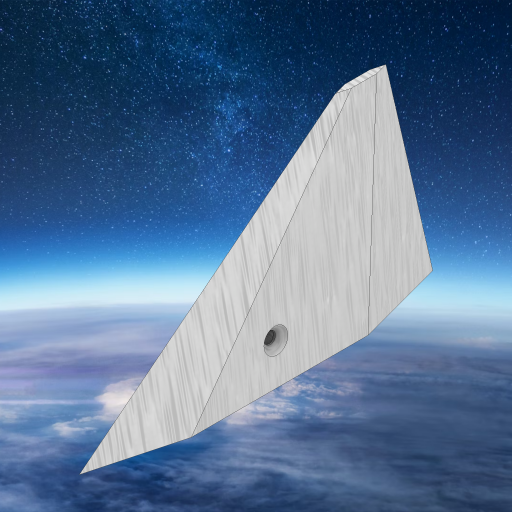
# Autodesk Inventor part: canard
Saved by Autodesk Inventor 2023 (Build 270158000, 158)
## iProperties
Created: 2022-11-29
Part Number: canard
Material: Aluminum 7075
Document SubType Name: Modeling
Designer: 310611102
Density: 2.81 g/cm^3
Appearance: Satin - Brushed Heavy
Mass: 264.064 g
Surface Area: 174.305 cm^2
Volume: 93.9731 cm^3
Author: 310611102
Autodesk Inventor part; units mm, degrees
ref_plane "XY Plane" through (0, 0, 0) normal (0, 0, 1) x (1, 0, 0)
sketch "草圖1" plane through (0, 0, 0) normal (1, 0, 0) x (0, 1, 0)
  line L0 (0, 0) -> (0, -140)
  line L1 (0, -140) -> (80, -121.4423)
  line L2 (80, -121.4423) -> (80, -101.4423)
  line L3 (80, -101.4423) -> (0, 0)
  line L4 (-21.2222, 0) -> (127.3329, 0) projected
  line L5 (0, -140) -> (106.1108, -140)
  dimension "d0" = 80
  dimension "d1" = 140
  dimension "d4" = 20
  dimension "d5" = 51.74
  dimension "d38" = 13.06
  constraints: 10 end point, 1 horizontal, 1 parallel, 1 vertical
  measures "d0" distance between parallel lines of L0 L2
  measures "d1" distance of L0.start L0.end
  measures "d4" distance of L1.end L2.end
  measures "d5" angle of L4 L3
  measures "d38" angle of L5 L1
sketch "草圖2" plane through (0, 0, 0) normal (0, 1, 0) x (-1, 0, 0)
  line L0 (0, -164.5545) -> (0, 20.7772)
  line L1 (0, 0) -> (9.3782, -35)
  line L2 (9.3782, -35) -> (9.3782, -105)
  line L3 (9.3782, -105) -> (0, -140)
  line L4 (0, -140) -> (-9.3782, -105)
  line L5 (-9.3782, -105) -> (-9.3782, -35)
  line L6 (-9.3782, -35) -> (0, 0)
  point P0 (9.3782, -70)
  point P1 (-9.3782, -70)
  dimension "d34" = 140
  dimension "d35" = 70
  dimension "d63" = 30
  constraints: 14 end point, 3 equal length, 2 midpoint, 2 vertical, 1 coincident, 1 parallel, 1 point on line, 1 other
  measures "d34" distance of L3.end point (0, 0)
  measures "d35" distance of L1.end L2.end
  measures "d63" angle of L1 L6
ref_plane "工作平面1" through (0, 40, 0) normal (0, 1, 0) x (-1, 0, 0)
sketch "草圖3" plane through (0, 40, 0) normal (0, 1, 0) x (-1, 0, 0)
  line L0 (0, -140) -> (0, -121.4423) construction
  line L1 (0, -101.4423) -> (0, 0) construction
  arc A0 (0, -130.7211) -> (0, -50.7211) centre (-157.5, -90.7211) ccw
  arc A1 (0, -50.7211) -> (0, -130.7211) centre (157.5, -90.7211) ccw
  point P0 (-5, -90.7211)
  point P1 (5, -90.7211)
  dimension "d8" = 10
  constraints: 6 point on circle, 4 midpoint, 2 centre point, 1 symmetric about line, 1 other
  measures "d8" distance of point (-5, -90.721) point (5, -90.721)
ref_plane "工作平面2" through (0, 80, -121.4423) normal (0, 1, 0) x (0, 0, 1)
sketch "草圖4" plane through (0, 80, -121.4423) normal (0, 1, 0) x (0, 0, 1)
  line L0 (0, 0) -> (20, 0) construction
  line L1 (0, 0) -> (5, -1.3397)
  line L2 (5, -1.3397) -> (15, -1.3397)
  line L3 (15, -1.3397) -> (20, 0)
  line L4 (20, 0) -> (15, 1.3397)
  line L5 (15, 1.3397) -> (5, 1.3397)
  line L6 (5, 1.3397) -> (0, 0)
  line L7 (0, 0) -> (23.7268, 0)
  point P0 (121.4423, 0)
  point P1 (10, 1.3397)
  point P2 (10, -1.3397)
  dimension "d36" = 20
  dimension "d37" = 10
  dimension "d62" = 30
  constraints: 14 end point, 2 equal length, 2 horizontal, 2 midpoint, 2 parallel, 1 coincident, 1 other
  measures "d36" distance of point (20, 0) L0.start
  measures "d37" distance of L1.end L2.end
  measures "d62" angle of L4 L3
loft "Loft3" add profiles "草圖4", "草圖2"
sketch "草圖5" plane through (0, 0, 0) normal (0, 1, 0) x (-1, 0, 0)
  circle A0 centre (0, -70) radius 5.1
  line L0 (0, -168) -> (0, 28) projected
  line L1 (-220.5, 0) -> (220.5, 0) projected
  point P0 (0, 0)
  dimension "d17" = 10.2
  dimension "d18" = 70
  constraints: 1 centre point, 1 midpoint
  measures "d17" diameter of A0
  measures "d18" distance from line of L1 A0.centre
extrude "擠出1" cut sketch "草圖5" along normal blind 20
sketch "Sketch12" plane through (9.3782, 0, -35) normal (0.9949897, 0.0999775, 0) x (0, 0, -1)
  line L0 (0, 0) -> (70, 0) projected
  line L1 (35, 0) -> (35, 15)
  point P0 (-35, 0.9376)
  dimension "d69" = 15
  constraints: 2 end point, 1 coincident, 1 midpoint, 1 vertical
  measures "d69" distance of L1.start L1.end
hole "Hole3" at (7.8786, 14.9248, -70) direction (-0.9949897, -0.0999775, 0) diameter 4.5 depth 10 tip angle 118 countersink diameter 9.4 countersink angle 90 clearance for "Countersunk Flat Head Screw ISO 2009/7046" size "M4" standard "ISO"
sketch "Sketch9" plane through (9.3782, 0, -35) normal (0.9949897, 0.0999775, 0) x (0, 0, -1)
  line L0 (86.4423, 80.5368) -> (105, 0.9376) projected
  line L1 (66.4423, 80.5368) -> (71.4423, 80.4028) projected
  line L2 (71.4423, 80.4028) -> (81.4423, 80.4028) projected
  line L3 (81.4423, 80.4028) -> (86.4423, 80.5368) projected
  line L4 (66.4423, 80.5368) -> (-35, 0.9376) projected
  line L5 (-35, 0.9376) -> (0, 0) projected
  line L6 (0, 0) -> (70, 0) projected
  line L7 (70, 0) -> (105, 0.9376) projected
sketch "Sketch7" plane through (9.3782, 0, -35) normal (0.9949897, 0.0999775, 0) x (0, 0, -1)
  line L0 (0, 0) -> (70, 0) projected
  line L1 (0, 0) -> (70, 0) projected
  line L2 (40, 0) -> (30, 0) projected
  line L3 (71.4423, 80.4028) -> (66.4423, 80.5368) projected
  line L4 (66.4423, 80.5368) -> (-35, 0.9376) projected
  line L5 (105, 0.9376) -> (86.4423, 80.5368) projected
  line L6 (71.4423, 80.4028) -> (81.4423, 80.4028) projected
  line L7 (-35, 0.9376) -> (0, 0) projected
  line L8 (70, 0) -> (105, 0.9376) projected
  line L9 (86.4423, 80.5368) -> (81.4423, 80.4028) projected
  point P0 (35, 15)
  dimension "d39" = 15
  measures "d39" distance from line of L0 point (35, 15)
sketch "Sketch8" plane through (9.3782, 0, -35) normal (0.9949897, 0.0999775, 0) x (0, 0, -1)
  circle A0 centre (55, 40) radius 2
  line L0 (0, 0) -> (70, 0) projected
  point P0 (-35, 0.9376)
  dimension "d49" = 40
  dimension "d50" = 90
  dimension "d51" = 4
  constraints: 1 centre point
  measures "d49" distance from line of L0 A0.centre
  measures "d50" horizontal distance of point (-35, 0.938) A0.centre
  measures "d51" diameter of A0
equation "\"d35\" = 0.5 * d34"
equation "\"d37\" = 0.5 * d36"
body "Solid3"
